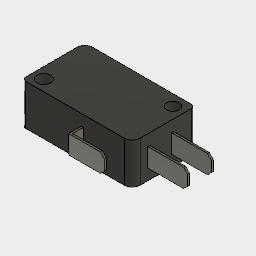
817 micro switch ZIPPY (Autodesk Fusion 360 design; units mm, degrees)
Autodesk Fusion 360 part; units mm, degrees
sketch "Sketch1" plane through (0, 0, 0) normal (0, 0, 1) x (1, 0, 0)
  line L0 (0, 0) -> (27.8, 0)
  line L1 (27.8, 0) -> (27.8, 15.9)
  line L2 (27.8, 15.9) -> (0, 15.9)
  line L3 (0, 15.9) -> (0, 0)
  circle A0 centre (2.8, 2.8) radius 1.7
  circle A1 centre (25, 13.1) radius 1.55
  line L4 (3.4, 15.9) -> (6.2, 15.9)
  line L5 (6.2, 15.9) -> (6.2, 18.9)
  line L6 (6.2, 18.9) -> (3.4, 18.9)
  line L7 (3.4, 18.9) -> (3.4, 15.9)
  line L8 (4.8, 18.9) -> (4.8, 15.9) construction
  line L9 (15, 0) -> (15, -3.2)
  line L10 (15, -3.2) -> (24, -3.2)
  line L11 (24, -3.2) -> (24, -2.7)
  line L12 (24, -2.7) -> (15.5, -2.7)
  line L13 (15.5, -2.7) -> (15.5, 0)
  line L14 (27.8, 10.45) -> (37.8, 10.45)
  line L15 (37.8, 10.45) -> (37.8, 9.95)
  line L16 (37.8, 9.95) -> (27.8, 9.95)
  line L17 (27.8, 9.95) -> (27.8, 10.45)
  line L18 (27.8, 4.45) -> (37.8, 4.45)
  line L19 (37.8, 4.45) -> (37.8, 3.95)
  line L20 (37.8, 3.95) -> (27.8, 3.95)
  line L21 (27.8, 3.95) -> (27.8, 4.45)
  dimension "d1" = 27.8
  dimension "d2" = 15.9
  dimension "d3" = 3.4
  dimension "d4" = 2.8
  dimension "d5" = 2.8
  dimension "d6" = 3.1
  dimension "d7" = 22.2
  dimension "d8" = 10.3
  dimension "d13" = 2.8
  dimension "d14" = 20.2
  dimension "d15" = 3
  dimension "d20" = 0.5
  dimension "d21" = 0.5
  dimension "d22" = 12.2
  dimension "d23" = 10
  dimension "d24" = 0.5
  dimension "d25" = 2.7
  dimension "d26" = 10
  dimension "d27" = 0.5
  dimension "d28" = 5.5
  dimension "d30" = 7.15
  dimension "d34" = 9
  measures "d1" distance of L0.start L0.end
  measures "d2" distance of L0.start L2.end
  measures "d3" diameter of A0
  measures "d4" distance of L0 A0.centre
  measures "d5" distance of L3 A0.centre
  measures "d6" diameter of A1
  measures "d7" distance of A0.centre A1.centre
  measures "d8" distance of A0.centre A1.centre
  measures "d13" distance of L5.end L6.end
  measures "d14" distance of A1.centre L8
  measures "d15" distance of L2 L6
  measures "d20" distance of L9 L13
  measures "d21" distance of L10 L12
  measures "d22" distance of A0.centre L9
  measures "d23" distance of L14.start L14.end
  measures "d24" distance of L14.start L16.end
  measures "d25" distance of L0 L12
  measures "d26" distance of L18.start L18.end
  measures "d27" distance of L18.start L20.end
  measures "d28" distance of L16 L18
  measures "d30" distance of L12 L18
  measures "d34" distance of L9 L11
extrude "Extrude1" add sketch "Sketch1" along normal blind 10.3 contours L0 L1 L2 L3 L4 L17 L21 makes body 1
fillet "Fillet1" radius 1 2 edges at (0, 0, 5.15) (27.8, 15.9, 5.15) on bodies 1
fillet "Fillet2" radius 2 2 edges at (27.8, 0, 5.15) (0, 15.9, 5.15) on bodies 1
ref_plane "WorkPlane1" through (13.9, 7.95, 5.15) normal (0, 0, 1) x (1, 0, 0)
extrude "Extrude2" add sketch "Sketch1" along normal mid plane 4.2 from surface at 5.15 contours L2 L4 L5 L6 L7 bodies 1
fillet "Fillet3" radius 1.4 2 edges at (3.4, 18.9, 5.15) (6.2, 18.9, 5.15) on bodies 1
extrude "Extrude3" add sketch "Sketch1" along normal mid plane 4.7 from surface at 5.15 separate body contours L0 L9 L10 L11 L12 L13 | L1 L18 L19 L20 L21 | L1 L14 L15 L16 L17 makes body 2 at (21, -3.2, 5.9333) makes body 3 at (34.4667, 3.95, 4.3667) makes body 4 at (31.1333, 10.45, 4.3667)
chamfer "Chamfer1" distance 1 angle 45 6 edges at (24, -2.95, 7.5) (24, -2.95, 2.8) (37.8, 10.2, 7.5) (37.8, 4.2, 7.5) (37.8, 10.2, 2.8) (37.8, 4.2, 2.8) on bodies 2 3 4
sketch "Sketch3" plane through (0, 0, 0) normal (0, 0, 1) x (1, 0, 0) in component "Component"
  line L0 (-3, 18.9) -> (30.8, 18.9)
  line L1 (30.8, 18.9) -> (30.8, -3)
  line L2 (30.8, -3) -> (-3, -3)
  line L3 (-3, -3) -> (-3, 18.9)
  line L4 (27.8, 2) -> (27.8, 14.9) construction
  line L5 (0, 13.9) -> (0, 1) construction
  line L6 (1, 0) -> (25.8, 0) construction
  line L7 (26.8, 15.9) -> (2, 15.9) construction
  circle A0 centre (25, 13.1) radius 1.55
  circle A1 centre (2.8, 2.8) radius 1.7
  circle A2 centre (2.8, 2.8) radius 3.2
  circle A3 centre (25, 13.1) radius 3.05
  dimension "d36" = 3
  dimension "d37" = 3
  dimension "d38" = 3
  dimension "d39" = 3
  dimension "d42" = 1.5
  dimension "d43" = 1.5
  measures "d36" distance of L1 L4
  measures "d37" distance of L3 L5
  measures "d38" distance of L2 L6
  measures "d39" distance of L0 L7
extrude "Extrude1'" add sketch "Sketch3" along normal blind 1 separate body contours L0 L1 L2 L3 | A2 | A3 makes body 5 in component "Component"
extrude "Extrude2'" add sketch "Sketch3" along normal blind 3 from surface at 1 contours A2 | A3 bodies 5 in component "Component"
chamfer "Chamfer1'" distance 1 angle 45 4 edges at (1.215, 3.4147, 0) (23.5549, 13.6605, 0) (-0.1834, 3.9572, 1) (22.1564, 14.2029, 1) on bodies 5 in component "Component"
fillet "Fillet1'" radius 2 4 edges at (-3, -3, 0.5) (-3, 18.9, 0.5) (30.8, 18.9, 0.5) (30.8, -3, 0.5) on bodies 5 in component "Component"
component "Component" placed x (1, 0, 0) y (0, 1, 0) z (0, 0, 1) at (0, 0, 0)
equation "d17 = ( 4.2 / 2 ) * 1 mm"
equation "d32 = ( 4.7 / 2 ) * 1 mm"
named bodies: "body", "Common 1", "NO 3", "NC 2"
